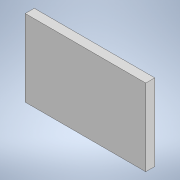
# Autodesk Inventor part: Sides_2
Saved by Autodesk Inventor 2020 (Build 240168000, 168)
## iProperties
Created: 2021-02-07
Part Number: Sides_2
Material: Generic
Document SubType Name: Modeling
Designer: moham
Density: 1 g/cm^3
Appearance: Default
Author: moham
Autodesk Inventor part; units mm, degrees
ref_plane "YZ Plane" through (0, 0, 0) normal (1, 0, 0) x (0, 1, 0)
ref_plane "XZ Plane" through (0, 0, 0) normal (0, 1, 0) x (-1, 0, 0)
ref_plane "XY Plane" through (0, 0, 0) normal (0, 0, 1) x (1, 0, 0)
sketch "Sketch1" plane through (0, 0, 0) normal (0, 0, 1) x (1, 0, 0)
  line L0 (-40, 25.5) -> (40, 25.5)
  line L1 (40, 25.5) -> (40, -25.5)
  line L2 (40, -25.5) -> (-40, -25.5)
  line L3 (-40, -25.5) -> (-40, 25.5)
  line L4 (-40, 25.5) -> (40, -25.5) construction
  line L5 (40, 25.5) -> (-40, -25.5) construction
  point P0 (0, 0)
  dimension "d2" = 51
  dimension "d3" = 80
  constraints: 12 end point, 2 midpoint, 2 parallel, 1 horizontal, 1 perpendicular
  measures "d2" distance of L0.end L1.end
  measures "d3" distance of L1.end L2.end
extrude "Extrusion1" add sketch "Sketch1" along normal blind 6
body "Solid1"
